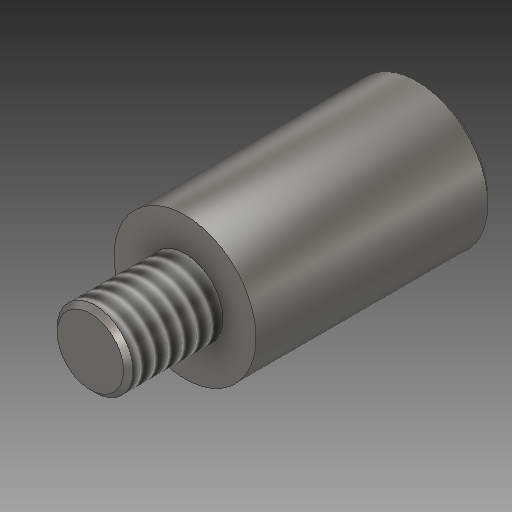
# Autodesk Inventor part: Perno tendi motore
Saved by Autodesk Inventor 2018 (Build 220112000, 112)
## iProperties
Created: 2020-06-04
Part Number: Perno tendi motore
Material: Acciaio inossidabile
Document SubType Name: Modeling
Designer: Francesco
Density: 8 g/cm^3
Appearance: Semilucidato
Mass: 39.294 g
Surface Area: 17.6104 cm^2
Volume: 4.91175 cm^3
Author: Francesco
Autodesk Inventor part; units mm, degrees
ref_plane "YZ Plane" through (0, 0, 0) normal (1, 0, 0) x (0, 1, 0)
ref_plane "XZ Plane" through (0, 0, 0) normal (0, 1, 0) x (-1, 0, 0)
ref_plane "XY Plane" through (0, 0, 0) normal (0, 0, 1) x (1, 0, 0)
sketch "Schizzo1" plane through (0, 0, 0) normal (0, 0, 1) x (1, 0, 0)
  circle A0 centre (0, 0) radius 7.5
  dimension "d0" = 15
  constraints: 1 centre point, 1 coincident
  measures "d0" diameter of A0
extrude "Estrusione1" add sketch "Schizzo1" along normal blind 25
sketch "Schizzo2" plane through (0, 0, 25) normal (0, 0, 1) x (1, 0, 0)
  circle A0 centre (0, 0) radius 4
  dimension "d3" = 8
  constraints: 1 centre point, 1 coincident
  measures "d3" diameter of A0
extrude "Estrusione2" add sketch "Schizzo2" along normal blind 10
chamfer "Smusso1" distance 0.5 angle 45 2 edges at (-4, 0, 35) (-7.5, 0, 0)
thread "Filettatura2" size "M10x1.5" class "6g" standard "ANSI Metric M Profile" full length
